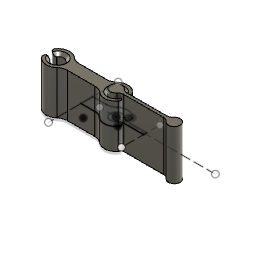
chain v2 (Autodesk Fusion 360 design; units mm, degrees)
Autodesk Fusion 360 part; units mm, degrees
sketch "Sketch1" plane through (0, 0, 0) normal (0, 1, 0) x (1, 0, 0)
  line L0 (0, 0) -> (34.1238, 0) construction
  line L1 (10, 5.0604) -> (10, -8.153) construction
  line L2 (3.1225, 0.5) -> (10, 0.5)
  line L3 (3.1225, -0.5) -> (10, -0.5)
  arc A0 (1.5612, 1.25) -> (1.5612, -1.25) centre (0, 0) ccw
  arc A1 (1.5612, 1.25) -> (3.1225, 0.5) centre (3.1225, 2.5) ccw
  arc A2 (3.1225, -0.5) -> (1.5612, -1.25) centre (3.1225, -2.5) ccw
  line L4 (2.3873, 1.8197) -> (0, 0) construction
  line L5 (0, 0) -> (-5.6498, 0) construction
  arc A3 (3.1812, 2.4249) -> (-2.6458, 3) centre (0, 0) ccw
  arc A4 (1.6545, 1.1417) -> (3.1812, 2.4249) centre (2.3873, 1.8197) ccw
  arc A5 (-2.6458, -3) -> (3.1812, -2.4249) centre (0, 0) ccw
  arc A6 (3.1812, -2.4249) -> (1.6545, -1.1417) centre (2.3873, -1.8197) ccw
  line L6 (-10, 10.7206) -> (-10, -13.2526) construction
  line L7 (-10, 2) -> (-5.2915, 2)
  line L8 (-10, -2) -> (-5.2915, -2)
  arc A7 (-5.2915, 2) -> (-2.6458, 3) centre (-5.2915, 6) ccw
  arc A8 (-2.6458, -3) -> (-5.2915, -2) centre (-5.2915, -6) ccw
  line L9 (10, 0.5) -> (10, -0.5)
  line L10 (-10, 2) -> (-10, -2)
  dimension "d1" = 4
  dimension "d2" = 10
  dimension "d3" = 0.5
  dimension "d4" = 0.5
  dimension "d5" = 2
  dimension "d6" = 8
  dimension "d7" = 37.316
  dimension "d8" = 10
  dimension "d9" = 2
  dimension "d10" = 2
  dimension "d11" = 4
  constraint coincident L0.start A0.centre
  constraint horizontal L0
  constraint vertical L1
  constraint coincident L1 L2.end
  constraint perpendicular L1 L2
  constraint coincident L1 L3.end
  constraint perpendicular L1 L3
  constraint tangent L2 A1
  constraint tangent A0 A1
  constraint tangent L3 A2
  constraint tangent A0 A2
  constraint equal A1 A2
  constraint concentric A0 A3
  constraint tangent A1 A4
  constraint tangent A3 A4
  constraint coincident L4.start A4.centre
  constraint parallel L0 L5
  constraint symmetric L0 A3 A5
  constraint symmetric L0 A3.start A5.end
  constraint symmetric L0 A4 A6
  constraint vertical L6
  constraint coincident L6 L7.start
  constraint perpendicular L6 L7
  constraint coincident L6 L8.start
  constraint perpendicular L6 L8
  constraint tangent L7 A7
  constraint tangent A3 A7
  constraint tangent L8 A8
  constraint tangent A5 A8
  constraint equal A7 A8
  constraint coincident A2 A6.end
  constraint coincident A1 A4.start
  measures "d1" diameter of A0
  measures "d2" distance of L0.start L1
  measures "d3" distance of L0 L2
  measures "d4" distance of L0 L3
  measures "d5" radius of A1
  measures "d6" diameter of A3
  measures "d7" angle of L0 L4
  measures "d8" distance of L0.start L6
  measures "d9" distance of L5 L7
  measures "d10" distance of L5 L8
  measures "d11" radius of A7
extrude "Extrude1" add sketch "Sketch1" along normal mid plane 17 contours L2 L3 A0 A1 A2 L9 makes body 1
extrude "Extrude2" add sketch "Sketch1" along normal mid plane 15 separate body contours A0 A1 A2 A3 A4 A5 A6 L7 L8 A7 A8 L10 makes body 2
chamfer "Chamfer1" distance 1 angle 45 2 edges at (-2, -7.5, 0) (-2, 7.5, 0) tangent chain off on bodies 2
mirror "Mirror1" about plane through (-10, 0, -2) normal (-1, 0, 0) of bodies 2 merged
mirror "Mirror2" about plane through (10, 0, -0.5) normal (1, 0, 0) of bodies 1 merged
named bodies: "chain flex", "chain asa"
